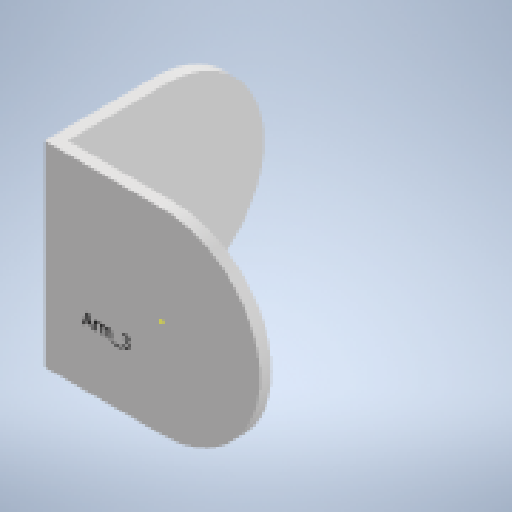
# Autodesk Inventor part: Arm_3
Saved by Autodesk Inventor 2023 (Build 270158000, 158)
## iProperties
Created: 2022-04-08
Part Number: Arm_3
Material: 一般
Document SubType Name: Modeling
Designer: device
Density: 1 g/cm^3
Appearance: 預設
Author: device
Autodesk Inventor part; units mm, degrees
ref_plane "XZ Plane" through (0, 0, 0) normal (0, 1, 0) x (-1, 0, 0)
ref_plane "XY Plane" through (0, 0, 0) normal (0, 0, 1) x (1, 0, 0)
sketch "草圖1" plane through (0, 0, 0) normal (0, 0, 1) x (1, 0, 0)
  line L0 (0, 0) -> (-100, 0) construction
  line L1 (0, 25) -> (-100, 25)
  line L2 (-100, -25) -> (0, -25)
  arc A0 (0, -25) -> (0, 25) centre (0, 0) ccw
  arc A1 (-100, 25) -> (-100, -25) centre (-100, 0) ccw
  circle A2 centre (0, 0) radius 25
  line L3 (-50, 25) -> (-55, 25)
  line L4 (-55, 25) -> (-55, -25)
  line L5 (-55, -25) -> (-50, -25)
  line L6 (-50, -25) -> (-50, 25)
  point P0 (-50, 0)
  point P1 (25, 0)
  point P2 (-125, 0)
  point P3 (-55, 25)
  dimension "d0" = 50
  dimension "d1" = 150
  dimension "d2" = 5
  constraints: 16 end point, 6 point on circle, 4 tangent, 3 parallel, 2 centre point, 2 horizontal, 2 midpoint, 1 coincident, 1 perpendicular, 1 point on line, 3 other
  measures "d0" diameter of A1
  measures "d1" distance of point (25, 0) point (-125, 0)
  measures "d2" distance between parallel lines of L4 L6
extrude "擠出1" add sketch "草圖1" along normal mid plane 3 contours A0 A2
sketch "草圖4" plane through (0, 0, 1.5) normal (0, 0, 1) x (1, 0, 0)
  line L0 (-20.1381, -7.4684) -> (-4.1343, -7.4684) construction
  line L1 (-4.1343, -7.4684) -> (-4.1343, -17.6042) construction
  line L2 (-4.1343, -17.6042) -> (-20.1381, -17.6042) construction
  line L3 (-20.1381, -17.6042) -> (-20.1381, -7.4684) construction
  point P0 (0, 0)
  constraints: 2 other
sketch "草圖5" plane through (0, 0, -1.5) normal (0, 0, -1) x (-1, 0, 0)
  circle A0 centre (0, 0) radius 25
  circle A1 centre (0, 0) radius 22
  dimension "d10" = 3
  constraints: 2 centre point, 1 coincident
  measures "d10" radial gap between concentric circles of A0 A1
extrude "擠出4" add sketch "草圖5" along normal blind 41
ref_plane "工作平面1" through (-25, 0, 0) normal (1, 0, 0) x (0, 1, 0)
sketch "草圖6" plane through (-25, 0, 0) normal (1, 0, 0) x (0, 1, 0)
  line L0 (-25, -42.5) -> (25, -42.5) construction
  line L1 (25, 1.5) -> (-25, 1.5) construction
  line L2 (-25, -42.5) -> (25, -42.5) construction
  line L3 (0, -42.5) -> (0, 1.5) construction
  line L4 (25, 1.5) -> (-25, 1.5) construction
  circle A0 centre (0, -20.5) radius 22
  point P0 (0, 0)
  constraints: 3 midpoint, 2 end point, 1 vertical alignment, 2 other
extrude "擠出5" add sketch "草圖6" along normal up to surface round surface about axis through (0, 0, -1.5) along (0, 0, -1) radius 22 far side no
